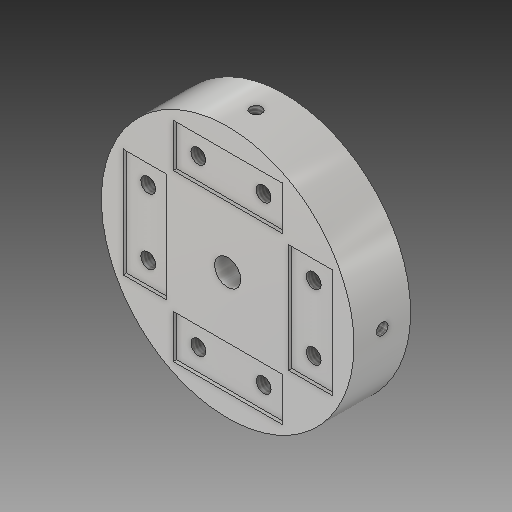
# Autodesk Inventor part: Bottom
Saved by Autodesk Inventor 2017 (Build 210142000, 142)
## iProperties
Created: 2016-06-22
Part Number: Bottom
Material: Generic
Document SubType Name: Modeling
Designer: Andres
Density: 1 g/cm^3
Appearance: Aluminum - Polished
Mass: 32.3763 g
Surface Area: 90.2787 cm^2
Volume: 32.3763 cm^3
Author: Andres
Autodesk Inventor part; units mm, degrees
ref_plane "YZ Plane" through (0, 0, 0) normal (1, 0, 0) x (0, 1, 0)
sketch "Sketch1" plane through (0, 0, 0) normal (0, 0, 1) x (1, 0, 0)
  circle A0 centre (0, 0) radius 29
  dimension "d0" = 58
  constraints: 1 centre point, 1 coincident
  measures "d0" diameter of A0
extrude "Extrusion1" add sketch "Sketch1" along normal blind 13
sketch "Sketch4" plane through (0, 0, 13) normal (0, 0, 1) x (1, 0, 0)
  circle A0 centre (0, 0) radius 3
  dimension "d7" = 6
  constraints: 1 centre point, 1 coincident
  measures "d7" diameter of A0
extrude "Extrusion3" cut sketch "Sketch4" against normal blind 13
ref_plane "Work Plane1" through (0, 0, 13) normal (0, 0, 1) x (1, 0, 0)
sketch "Sketch10" plane through (0, 0, 13) normal (0, 0, 1) x (1, 0, 0)
  point P0 (0, 0)
sketch "Sketch11" plane through (0, 0, 13) normal (0, 0, 1) x (1, 0, 0)
  circle A0 centre (0, 0) radius 3 projected
  line L0 (-12.5, 14) -> (12.5, 14)
  line L1 (12.5, 14) -> (12.5, 24)
  line L2 (12.5, 24) -> (-12.5, 24)
  line L3 (-12.5, 24) -> (-12.5, 14)
  point P0 (0, 14)
  point P1 (-7.5, 19)
  point P2 (7.5, 19)
  dimension "d54" = 25
  dimension "d55" = 14
  dimension "d56" = 10
  dimension "d57" = 5
  dimension "d58" = 5
  dimension "d59" = 5
  dimension "d60" = 5
  constraints: 8 end point, 2 perpendicular, 1 horizontal, 1 midpoint, 1 vertical, 1 vertical alignment
  measures "d54" distance of L0.start L0.end
  measures "d55" distance from line of L0 point (0, 0)
  measures "d56" distance of L0.end L1.end
  measures "d57" distance from line of L3 point (-7.5, 19)
  measures "d58" distance from line of L1 point (7.5, 19)
  measures "d59" distance from line of L0 point (7.5, 19)
  measures "d60" distance from line of L0 point (-7.5, 19)
hole "Hole2" at (-7.5, 19, 13) at (7.5, 19, 13) direction (0, 0, -1) diameter 3.404 depth 12 thread size "8-36 UNF" class "2B" standard "ANSI Unified Screw Threads"
extrude "Extrusion8" cut sketch "Sketch11" against normal blind 0.76 contours L3 L2 L1 L0
pattern_circular "Circular Pattern2" count 4 over 360 about axis through (0, 0, 13) along (0, 0, -1) of "Extrusion8", "Hole2"
ref_plane "Work Plane2" through (-12.5, -28.99998, 13) normal (0, -1, 0) x (1, 0, 0)
sketch "Sketch12" plane through (-12.5, -28.99998, 13) normal (0, -1, 0) x (1, 0, 0)
  point P0 (12.5, -13)
  point P1 (12.5, -6.5)
  dimension "d74" = 6.5
  constraints: 1 vertical alignment
  measures "d74" distance of point (12.5, -6.5) point (12.5, -13)
hole "Hole3" at (0, -28.99998, 6.5) direction (0, 1, 0) diameter 2.642 depth 58 tip angle 118 thread size "6-32 UNC" class "3B" standard "ANSI Unified Screw Threads"
pattern_circular "Circular Pattern3" count 2 over 90 about axis through (0, 0, 13) along (0, 0, -1) of "Hole3"
body "Solid1"
